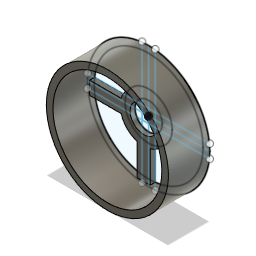
dc-15s_led_assembly (Autodesk Fusion 360 design; units mm, degrees)
Autodesk Fusion 360 part; units mm, degrees
sketch "Sketch1" plane through (0, 0, 0) normal (0, 0, 1) x (1, 0, 0)
  circle A0 centre (0, 0) radius 18.5
  circle A1 centre (0, 0) radius 4.125
  circle A2 centre (0, 0) radius 16.5
  line L0 (-18.5, 0) -> (18.5, 0)
  line L1 (0, 18.5) -> (0, -18.5)
  line L2 (-18.5, 2) -> (18.5, 2)
  line L3 (-18.5, -2) -> (18.5, -2)
  line L4 (-2, 18.5) -> (-2, -18.5)
  line L5 (2, 18.5) -> (2, -18.5)
  circle A3 centre (0, 0) radius 7.125
  dimension "d1" = 37
  dimension "d2" = 8.25
  dimension "d4" = -2
  dimension "d5" = -2
  dimension "d6" = 2
  dimension "d7" = 2
  dimension "d8" = -2
  dimension "d13" = 3
  constraint coincident A0.centre A1.centre
  constraint concentric A0 A1
  constraint coincident A0 L0.start
  constraint coincident A0 L0.end
  constraint horizontal L0
  constraint coincident A0 L1.start
  constraint coincident A0 L1.end
  constraint perpendicular L0 L1
  measures "d1" diameter of A0
  measures "d2" diameter of A1
extrude "Extrude2" add sketch "Sketch1" along normal blind 12.5 contours A0 A2 L0 L2 | A0 A2 L0 L3 | A0 A2 L2 L5 | A0 A2 L3 L5 | A0 A2 L1 L5 | A0 A2 L1 L5 | A0 A2 L1 L4 | A0 A2 L1 L4 | A0 A2 L2 L4 | A0 A2 L3 L4 | A0 A2 L0 L2 | A0 A2 L0 L3
extrude "Extrude1" add sketch "Sketch1" along normal blind 1.5 contours A0 A2 L0 L2 | A0 A2 L0 L3 | A2 L0 L2 A3 | A2 L0 L3 A3 | A0 A2 L1 L5 | A0 A2 L1 L5 | A1 L0 L3 A3 | A1 L0 L2 A3 | A2 L1 L5 A3 | A1 L2 L5 A3 | A0 A2 L1 L4 | A2 L1 L5 A3 | A1 L3 L5 A3 | A2 L1 L4 A3 | A1 L1 L5 A3 | A2 L1 L4 A3 | A1 L1 L5 A3 | A0 A2 L0 L2 | A1 L1 L4 A3 | A0 A2 L0 L3 | A1 L1 L4 A3 | A2 L0 L2 A3 | A1 L2 L4 A3 | A2 L0 L3 A3 | A1 L3 L4 A3 | A1 L0 L2 A3 | A1 L0 L3 A3 picked at (-1.7784, -17.0719)
